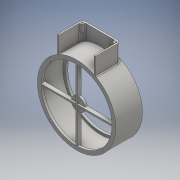
# Autodesk Inventor part: Motor mount (plain)
Saved by Autodesk Inventor 2016 (Build 200138000, 138)
## iProperties
Created: 2016-03-10
Part Number: Motor mount (plain)
Material: Generic
Document SubType Name: Modeling
Designer: s_sud
Density: 1 g/cm^3
Appearance: Default
Author: s_sud
Autodesk Inventor part; units mm, degrees
ref_plane "YZ Plane" through (0, 0, 0) normal (1, 0, 0) x (0, 1, 0)
ref_plane "XZ Plane" through (0, 0, 0) normal (0, 1, 0) x (-1, 0, 0)
sketch "Sketch1" plane through (0, 0, 0) normal (0, 1, 0) x (-1, 0, 0)
  circle A0 centre (0, 0) radius 50
  circle A1 centre (0, 0) radius 51.5
  dimension "d0" = 100
  dimension "d1" = 103
  constraints: 2 centre point, 2 coincident
  measures "d0" diameter of A0
  measures "d1" diameter of A1
extrude "Extrusion1" add sketch "Sketch1" along normal blind 35
sketch "Sketch12" plane through (0, 0, 0) normal (0, -1, 0) x (1, 0, 0)
  line L0 (-1, -51) -> (1, -51)
  line L1 (1, -51) -> (1, 51)
  line L2 (1, 51) -> (-1, 51)
  line L3 (-1, 51) -> (-1, -51)
  line L4 (-1, -51) -> (1, 51) construction
  line L5 (1, -51) -> (-1, 51) construction
  line L6 (-51, -1) -> (51, -1)
  line L7 (51, -1) -> (51, 1)
  line L8 (51, 1) -> (-51, 1)
  line L9 (-51, 1) -> (-51, -1)
  line L10 (-51, -1) -> (51, 1) construction
  line L11 (51, -1) -> (-51, 1) construction
  point P0 (0, 0)
  dimension "d64" = 102
  dimension "d65" = 2
  dimension "d66" = 102
  dimension "d67" = 2
  constraints: 24 end point, 4 midpoint, 4 parallel, 2 horizontal, 2 perpendicular
  measures "d64" distance of L0.end L1.end
  measures "d65" distance of L0.start L0.end
  measures "d66" distance of L7.end L8.end
  measures "d67" distance of L6.end L7.end
extrude "Extrusion12" add sketch "Sketch12" against normal blind 5
sketch "Sketch13" plane through (0, 5, 0) normal (0, 1, 0) x (1, 0, 0)
  circle A0 centre (0, 0) radius 9
  circle A1 centre (0, 6) radius 1
  circle A2 centre (-4.2426, 4.2426) radius 1
  circle A3 centre (-6, 0) radius 1
  circle A4 centre (-4.2426, -4.2426) radius 1
  circle A5 centre (0, -6) radius 1
  circle A6 centre (4.2426, -4.2426) radius 1
  circle A7 centre (6, 0) radius 1
  circle A8 centre (4.2426, 4.2426) radius 1
  dimension "d70" = 18
  dimension "d71" = 2
  dimension "d72" = 6
  dimension "d75" = 360
  constraints: 9 centre point, 1 coincident, 17 other
  measures "d70" diameter of A0
  measures "d71" diameter of A1
  measures "d72" distance of point (0, 0) A1.centre
extrude "Extrusion13" add sketch "Sketch13" against normal blind 3 contours A0 | A1 | A3 | A5 | A7
sketch "Sketch14" plane through (0, 0, 0) normal (0, -1, 0) x (1, 0, 0)
  circle A0 centre (0, 0) radius 46.5
  circle A1 centre (0, 0) radius 51.5
  dimension "d79" = 93
  dimension "d80" = 103
  constraints: 2 centre point, 2 coincident
  measures "d79" diameter of A0
  measures "d80" diameter of A1
extrude "Extrusion14" add sketch "Sketch14" against normal blind 3
sketch "Sketch15" plane through (0, 35, 0) normal (0, 1, 0) x (1, 0, 0)
  circle A0 centre (0, 0) radius 46.5
  circle A1 centre (0, 0) radius 51.5
  dimension "d83" = 93
  dimension "d84" = 103
  constraints: 2 centre point, 2 coincident
  measures "d83" diameter of A0
  measures "d84" diameter of A1
extrude "Extrusion15" add sketch "Sketch15" against normal blind 3
sketch "Sketch16" plane through (0, 35, 0) normal (0, 1, 0) x (1, 0, 0)
  circle A0 centre (0, 49) radius 1
  circle A1 centre (-34.6482, 34.6482) radius 1
  circle A2 centre (-49, 0) radius 1
  circle A3 centre (-34.6482, -34.6482) radius 1
  circle A4 centre (0, -49) radius 1
  circle A5 centre (34.6482, -34.6482) radius 1
  circle A6 centre (49, 0) radius 1
  circle A7 centre (34.6482, 34.6482) radius 1
  point P0 (0, 0)
  dimension "d87" = 2
  dimension "d88" = 49
  dimension "d91" = 360
  constraints: 8 centre point, 17 other
  measures "d87" diameter of A0
  measures "d88" distance of point (0, 0) A0.centre
extrude "Extrusion16" cut sketch "Sketch16" against normal blind 100 contours A1 | A3 | A5 | A7
ref_plane "Work Plane1" through (0, 0, 58) normal (0, 0, 1) x (1, 0, 0)
sketch "Sketch17" plane through (0, 0, 58) normal (0, 0, 1) x (1, 0, 0)
  line L0 (25, 0) -> (25, 28.1967)
  line L1 (20, 33.1967) -> (-20, 33.1967)
  line L2 (-25, 28.1967) -> (-25, 0)
  line L3 (-25, -33.1967) -> (25, 33.1967) construction
  line L4 (25, -33.1967) -> (-25, 33.1967) construction
  line L5 (46.4892, 0) -> (1, 0) projected
  line L6 (-23.2143, 0) -> (-23.2143, 25.8256)
  line L7 (-18.2143, 30.8256) -> (18.2143, 30.8256)
  line L8 (23.2143, 25.8256) -> (23.2143, 0)
  line L9 (23.2143, -30.8256) -> (-23.2143, 30.8256) construction
  line L10 (-23.2143, -30.8256) -> (23.2143, 30.8256) construction
  line L11 (-25, 0) -> (-23.2143, 0)
  line L12 (23.2143, 0) -> (25, 0)
  arc A0 (-18.2143, 30.8256) -> (-23.2143, 25.8256) centre (-18.2143, 25.8256) ccw
  arc A1 (23.2143, 25.8256) -> (18.2143, 30.8256) centre (18.2143, 25.8256) ccw
  arc A2 (25, 28.1967) -> (20, 33.1967) centre (20, 28.1967) ccw
  arc A3 (-20, 33.1967) -> (-25, 28.1967) centre (-20, 28.1967) ccw
  point P0 (0, 0)
  dimension "d96" = 50
  dimension "d101" = 5
  constraints: 24 end point, 10 point on line, 8 point on circle, 8 tangent, 4 centre point, 4 midpoint, 3 equal radius, 2 parallel
  measures "d96" distance of L4.end L3.end
  measures "d101" radius of A0
extrude "Extrusion17" add sketch "Sketch17" against normal blind 13 and the other way blind 10
fillet "Fillet2" radius 2 5 edges at (25, 14.0983, 45.025) (23.6885, 31.5723, 45.7286) (0, 33.1967, 51.5) (-23.684, 31.5772, 45.7309) (-25, 14.0983, 45.025)
sketch "Sketch19" plane through (0, 0, 68) normal (0, 0, 1) x (1, 0, 0)
  arc A0 (-18.2143, 30.8256) -> (-21.7945, 29.3159) centre (-18.2143, 25.8256) ccw projected
  circle A1 centre (-21.7945, 29.3159) radius 2.5
  circle A2 centre (21.9389, 29.3159) radius 2.5
  line L0 (-23.2143, 0) -> (23.2143, 0) projected
  point P0 (0, 0)
  dimension "d105" = 5
  dimension "d106" = 5
  dimension "d107" = 29.3159
  constraints: 2 centre point
  measures "d105" diameter of A2
  measures "d106" diameter of A1
  measures "d107" distance from line of L0 A1.centre
extrude "Extrusion18" add sketch "Sketch19" against normal blind 10
sketch "Sketch20" plane through (0, 0, 68) normal (0, 0, 1) x (1, 0, 0)
  arc A0 (-18.2143, 30.8256) -> (-21.7945, 29.3159) centre (-18.2143, 25.8256) ccw projected
  circle A1 centre (-21.7945, 29.3159) radius 1
  circle A2 centre (22.324, 29.3159) radius 1
  point P0 (0, 0)
  dimension "d110" = 2
  dimension "d111" = 2
  constraints: 2 centre point
  measures "d110" diameter of A1
  measures "d111" diameter of A2
extrude "Extrusion19" cut sketch "Sketch20" against normal blind 10
body "Solid1"
